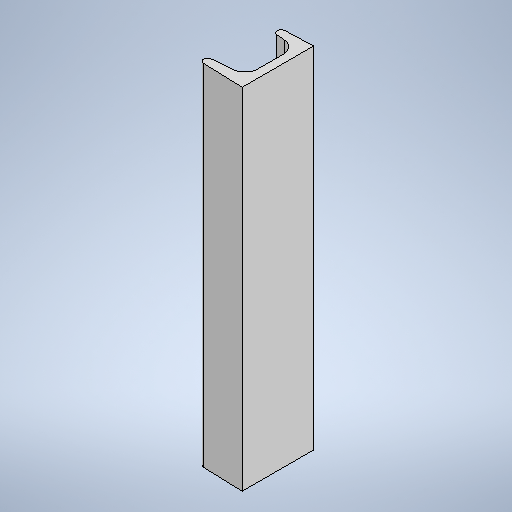
# Autodesk Inventor part: Bunk 1
Saved by Autodesk Inventor 2025 (Build 290162000, 162)
## iProperties
Created: 2026-03-19
Part Number: Bunk 1
Material: Generic
Document SubType Name: Modeling
Designer: steve
Density: 1 g/cm^3
Appearance: Default
Author: steve
Autodesk Inventor part; units mm, degrees
ref_plane "YZ Plane" through (0, 0, 0) normal (1, 0, 0) x (0, 1, 0)
ref_plane "XZ Plane" through (0, 0, 0) normal (0, 1, 0) x (-1, 0, 0)
ref_plane "XY Plane" through (0, 0, 0) normal (0, 0, 1) x (1, 0, 0)
sketch "Sketch1" plane through (0, 0, 0) normal (0, 1, 0) x (-1, 0, 0)
  line L0 (0, -675.5952) -> (0, 696.4048) construction
  line L1 (-230, 0) -> (610, 0) construction
  line L2 (0, 337.0036) -> (0, -337.0036)
  line L3 (0, -337.0036) -> (320, -365)
  line L4 (320, -365) -> (320, -464.5793)
  line L5 (0, 337.0036) -> (490, 379.8731)
  line L6 (490, 379.8731) -> (490, 479.4523)
  line L7 (490, 479.4523) -> (-110, 500.4048)
  line L8 (-110, 500.4048) -> (-110, -479.5952)
  line L9 (-110, -479.5952) -> (320, -464.5793)
  line L10 (320, -365) -> (320, 365) construction
  point P0 (0, 0)
  point P1 (320, -414.7896)
  dimension "d0" = 730
  dimension "d2" = 430
  dimension "d3" = 600
  dimension "d4" = 980
  dimension "d5" = 88
  dimension "d6" = 88
  dimension "d7" = 95
  dimension "d8" = 95
  dimension "d9" = 490
  constraints: 18 end point, 4 parallel, 3 point on line, 2 midpoint, 1 vertical
  measures "d0" distance of L3.end L10.end
  measures "d2" distance from line of point (320, -414.79) L8
  measures "d3" distance between parallel lines of L6 L8
  measures "d4" distance of L7.end L8.end
  measures "d5" angle of L8 L9
  measures "d6" angle of L8 L7
  measures "d7" angle of L2 L5
  measures "d8" angle of L3 L2
  measures "d9" distance between parallel lines of L6 L2
extrude "Extrusion1" add sketch "Sketch1" along normal mid plane 4800
fillet "Fillet1" radius 50 4 edges at (-320, 0, -464.5793) (-320, 0, -365) (-490, 0, 379.8731) (-490, 0, 479.4523)
fillet "Fillet2" radius 180 2 edges at (0, 0, 337.0036) (0, 0, -337.0036)
equation "\"d6\" = d5"
body "Solid1"
